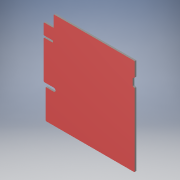
# Autodesk Inventor part: Avionics_PCB
Saved by Autodesk Inventor 2018 (Build 220112000, 112)
## iProperties
Created: 2018-01-15
Part Number: Avionics_PCB
Material: Epoxy Resin
Document SubType Name: Modeling
Designer: Bradley
Density: 1.14 g/cm^3
Appearance: Smooth - Medium Gray
Mass: 15.4834 g
Surface Area: 175.95 cm^2
Volume: 13.582 cm^3
Author: Bradley
Revision Number: 3.1
Autodesk Inventor part; units mm, degrees
ref_plane "XZ Plane" through (0, 0, 0) normal (0, 1, 0) x (-1, 0, 0)
ref_plane "XY Plane" through (0, 0, 0) normal (0, 0, 1) x (1, 0, 0)
sketch "Sketch1" plane through (0, 0, 0) normal (0, 0, 1) x (1, 0, 0)
  line L0 (0, 36.15) -> (10, 36.15)
  line L1 (10, 36.15) -> (10, 47.9)
  line L2 (10, 47.9) -> (90.4, 47.9)
  line L3 (90.4, 47.9) -> (90.4, -47.9)
  line L4 (90.4, -47.9) -> (2, -47.9)
  line L5 (10, -15.15) -> (0, -15.15)
  line L6 (-5.5, 48) -> (90.5, 48) construction
  line L7 (90.5, 48) -> (90.5, -48) construction
  line L8 (90.5, -48) -> (-5.5, -48) construction
  line L9 (-5.5, -48) -> (-5.5, 48) construction
  line L10 (-5.4, 47.9) -> (-3.4, 47.9) construction
  line L11 (-3.4, 47.9) -> (-3.4, -47.9) construction
  line L12 (-3.4, -47.9) -> (-5.4, -47.9) construction
  line L13 (-5.4, -47.9) -> (-5.4, 47.9) construction
  line L14 (-3.4, 38.5) -> (7.85, 38.5) construction
  line L15 (7.85, 38.5) -> (7.85, -17.5) construction
  line L16 (7.85, -17.5) -> (-3.4, -17.5) construction
  line L17 (-3.4, -17.5) -> (-3.4, 38.5) construction
  line L18 (2, -47.9) -> (2, -18.65)
  line L19 (2, -18.65) -> (10, -18.65)
  arc A0 (10, -18.65) -> (10, -15.15) centre (10, -16.9) ccw
  line L20 (0, 24) -> (90.5, 24) construction
  circle A1 centre (-2.5, 47.1) radius 0.9 construction
  circle A2 centre (-0.7, 47.1) radius 0.9 construction
  circle A3 centre (1.1, 47.1) radius 0.9 construction
  circle A4 centre (2.9, 47.1) radius 0.9 construction
  circle A5 centre (4.7, 47.1) radius 0.9 construction
  circle A6 centre (6.5, 47.1) radius 0.9 construction
  circle A7 centre (8.3, 47.1) radius 0.9 construction
  circle A8 centre (-2.5, 45.3) radius 0.9 construction
  circle A9 centre (-0.7, 45.3) radius 0.9 construction
  circle A10 centre (1.1, 45.3) radius 0.9 construction
  circle A11 centre (2.9, 45.3) radius 0.9 construction
  circle A12 centre (4.7, 45.3) radius 0.9 construction
  circle A13 centre (6.5, 45.3) radius 0.9 construction
  circle A14 centre (8.3, 45.3) radius 0.9 construction
  circle A15 centre (-2.5, 43.5) radius 0.9 construction
  circle A16 centre (-0.7, 43.5) radius 0.9 construction
  circle A17 centre (1.1, 43.5) radius 0.9 construction
  circle A18 centre (2.9, 43.5) radius 0.9 construction
  circle A19 centre (4.7, 43.5) radius 0.9 construction
  circle A20 centre (6.5, 43.5) radius 0.9 construction
  circle A21 centre (8.3, 43.5) radius 0.9 construction
  circle A22 centre (-2.5, 41.7) radius 0.9 construction
  circle A23 centre (-0.7, 41.7) radius 0.9 construction
  circle A24 centre (1.1, 41.7) radius 0.9 construction
  circle A25 centre (2.9, 41.7) radius 0.9 construction
  circle A26 centre (4.7, 41.7) radius 0.9 construction
  circle A27 centre (6.5, 41.7) radius 0.9 construction
  circle A28 centre (8.3, 41.7) radius 0.9 construction
  circle A29 centre (-2.5, 39.9) radius 0.9 construction
  circle A30 centre (-0.7, 39.9) radius 0.9 construction
  circle A31 centre (1.1, 39.9) radius 0.9 construction
  circle A32 centre (2.9, 39.9) radius 0.9 construction
  circle A33 centre (4.7, 39.9) radius 0.9 construction
  circle A34 centre (6.5, 39.9) radius 0.9 construction
  circle A35 centre (8.3, 39.9) radius 0.9 construction
  line L21 (0, 36.15) -> (0, 24.95)
  line L22 (0, 24.95) -> (8.4, 24.95)
  arc A36 (8.4, 23.05) -> (8.4, 24.95) centre (8.4, 24) ccw
  line L23 (8.4, 23.05) -> (0, 23.05)
  line L24 (0, 23.05) -> (0, -15.15)
  point P0 (0, 0)
  point P1 (-5.5, 0)
  point P2 (90.4, 0)
  point P3 (90.5, 0)
  dimension "d0" = 51.3
  dimension "d1" = 95.8
  dimension "d3" = 10
  dimension "d20" = 96
  dimension "d21" = 96
  dimension "d22" = 0.1
  dimension "d23" = 0.1
  dimension "d24" = 2
  dimension "d25" = 0.1
  dimension "d28" = 11.25
  dimension "d29" = 56
  dimension "d31" = 9.5
  dimension "d32" = 30.5
  dimension "d34" = 3.5
  dimension "d35" = 12.15
  dimension "d36" = 39.15
  dimension "d37" = 14.5
  dimension "d38" = 1.15
  dimension "d39" = 1.8
  dimension "d42" = 1.8
  dimension "d45" = 1.8
  dimension "d48" = 2
  dimension "d49" = 3.4
  dimension "d50" = 1.9
  dimension "d51" = 8.4
  dimension "d52" = 24
  constraints: 50 end point, 37 centre point, 11 perpendicular, 7 parallel, 6 point on line, 6 tangent, 5 horizontal, 4 point on circle, 3 midpoint, 3 vertical, 2 collinear, 2 horizontal alignment, 68 other
  measures "d0" distance of L5.end L0.start
  measures "d1" distance of L2.end L3.end
  measures "d3" distance of L0.start L0.end
  measures "d20" distance of L6.start L6.end
  measures "d21" distance of L8.end L6.start
  measures "d22" distance between parallel lines of L2 L6
  measures "d23" distance between parallel lines of L7 L3
  measures "d24" distance between parallel lines of L13 L11
  measures "d25" distance between parallel lines of L13 L9
  measures "d28" distance of L15.end L16.end
  measures "d29" distance of L14.end L15.end
  measures "d31" distance between parallel lines of L14 L6
  measures "d32" distance between parallel lines of L8 L16
  measures "d34" distance between parallel lines of L5 L19
  measures "d35" distance between parallel lines of L20 L0
  measures "d36" distance between parallel lines of L5 L20
  measures "d37" distance between parallel lines of L20 L14
  measures "d38" distance between parallel lines of L19 L16
  measures "d39" diameter of A1
  measures "d42" distance of A1.centre A2.centre
  measures "d45" distance of A1.centre A8.centre
  measures "d48" distance between parallel lines of L18 L24
  measures "d49" distance between parallel lines of L24 L11
  measures "d50" distance between parallel lines of L23 L22
  measures "d51" distance of L21.end L22.end
  measures "d52" distance from line of point (0, 0) L20
extrude "Extrusion1" add sketch "Sketch1" along normal mid plane 1.6
chamfer "Chamfer1" distance 0.5 angle 45 4 edges at (0, 36.15, 0) (0, 24.95, 0) (0, 23.05, 0) (0, -15.15, 0)
fillet "Fillet1" radius 0.5 6 edges at (10, 36.15, 0) (10, 47.9, 0) (90.4, 47.9, 0) (90.4, -47.9, 0) (2, -47.9, 0) (2, -18.65, 0)
sketch "Sketch16" plane through (0, 0, 0.8) normal (0, 0, 1) x (1, 0, 0)
  arc A0 (2.5, -18.65) -> (2, -19.15) centre (2.5, -19.15) ccw projected
  line L0 (2, -19.15) -> (2, -47.4) projected
  arc A1 (2, -47.4) -> (2.5, -47.9) centre (2.5, -47.4) ccw projected
  line L1 (2.5, -47.9) -> (89.9, -47.9) projected
  arc A2 (89.9, -47.9) -> (90.4, -47.4) centre (89.9, -47.4) ccw projected
  line L2 (90.4, -47.4) -> (90.4, 47.4) projected
  arc A3 (90.4, 47.4) -> (89.9, 47.9) centre (89.9, 47.4) ccw projected
  line L3 (89.9, 47.9) -> (10.5, 47.9) projected
  arc A4 (10.5, 47.9) -> (10, 47.4) centre (10.5, 47.4) ccw projected
  line L4 (10, 47.4) -> (10, 36.65) projected
  arc A5 (9.5, 36.15) -> (10, 36.65) centre (9.5, 36.65) ccw projected
  line L5 (9.5, 36.15) -> (0.5, 36.15) projected
  line L6 (0, 35.65) -> (0.5, 36.15) projected
  line L7 (0, 35.65) -> (0, 25.45) projected
  line L8 (0.5, 24.95) -> (0, 25.45) projected
  line L9 (0.5, 24.95) -> (8.4, 24.95) projected
  arc A6 (8.4, 23.05) -> (8.4, 24.95) centre (8.4, 24) ccw projected
  line L10 (8.4, 23.05) -> (0.5, 23.05) projected
  line L11 (0, 22.55) -> (0.5, 23.05) projected
  line L12 (0, 22.55) -> (0, -14.65) projected
  line L13 (0.5, -15.15) -> (0, -14.65) projected
  line L14 (0.5, -15.15) -> (10, -15.15) projected
  arc A7 (10, -18.65) -> (10, -15.15) centre (10, -16.9) ccw projected
  line L15 (10, -18.65) -> (2.5, -18.65) projected
  line L16 (90.4, -47.4) -> (90.4, 47.4) projected
  arc A8 (89.4, 33) -> (90.4, 34) centre (89.4, 34) ccw
  arc A9 (89.4, 33) -> (88.4, 32) centre (89.4, 32) ccw
  arc A10 (88.4, 26) -> (89.4, 25) centre (89.4, 26) ccw
  arc A11 (90.4, 24) -> (89.4, 25) centre (89.4, 24) ccw
  line L17 (88.4, 32) -> (88.4, 26)
  line L18 (88.4, 29) -> (90.4, 29) construction
  point P0 (0, 0)
  dimension "d145" = 1
  dimension "d146" = 29
  dimension "d147" = 8
  dimension "d148" = 34
  constraints: 8 point on circle, 6 tangent, 4 centre point, 4 end point, 3 equal radius, 3 point on line, 1 midpoint, 1 perpendicular, 1 vertical, 1 vertical alignment
  measures "d145" radius of A11
  measures "d146" distance from line of L18 point (0, 0)
  measures "d147" distance of A10.end A8.start
  measures "d148" vertical distance of point (0, 0) A8.end
extrude "Extrusion6" cut sketch "Sketch16" against normal through all contours A11 A10 L17 A9 A8 L2
ref_plane "Work Plane1" through (4, 0, 0) normal (1, 0, 0) x (0, 1, 0)
sketch "Sketch17" plane through (4, 0, 0) normal (1, 0, 0) x (0, 1, 0)
  line L0 (-19.15, -0.8) -> (-19.15, 0.8) projected
  line L1 (-47.4, -0.8) -> (-19.15, -0.8) projected
  line L2 (-47.4, 0.8) -> (-47.4, -0.8) projected
  line L3 (-19.15, 0.8) -> (-47.4, 0.8) projected
  point P0 (0, 0)
  point P1 (-42, 1.8)
  point P2 (-41, 1.8)
  point P3 (-40, 1.8)
  point P4 (-39, 1.8)
  point P5 (-42, 2.8)
  point P6 (-41, 2.8)
  point P7 (-40, 2.8)
  point P8 (-39, 2.8)
  point P9 (-42, 3.8)
  point P10 (-41, 3.8)
  point P11 (-40, 3.8)
  point P12 (-39, 3.8)
  point P13 (-42, 4.8)
  point P14 (-41, 4.8)
  point P15 (-40, 4.8)
  point P16 (-39, 4.8)
  dimension "d154" = 1
  dimension "d157" = 1
  dimension "d160" = 42
  dimension "d161" = 1
  constraints: 1 horizontal, 1 vertical, 15 other
  measures "d154" distance of point (-42, 1.8) point (-41, 1.8)
  measures "d157" distance of point (-42, 1.8) point (-42, 2.8)
  measures "d160" horizontal distance of point (-42, 1.8) point (0, 0)
  measures "d161" distance from line of L3 point (-42, 1.8)
sketch "Sketch18" plane through (0, 0, 0) normal (0, 0, 1) x (1, 0, 0)
  arc A0 (90.4, 24) -> (89.4, 25) centre (89.4, 24) ccw projected
  arc A1 (88.4, 26) -> (89.4, 25) centre (89.4, 26) ccw projected
  line L0 (88.4, 26) -> (88.4, 32) projected
  arc A2 (89.4, 33) -> (88.4, 32) centre (89.4, 32) ccw projected
  arc A3 (89.4, 33) -> (90.4, 34) centre (89.4, 34) ccw projected
  line L1 (90.4, 34) -> (90.4, 47.4) projected
  arc A4 (90.4, 47.4) -> (89.9, 47.9) centre (89.9, 47.4) ccw projected
  line L2 (89.9, 47.9) -> (10.5, 47.9) projected
  arc A5 (10.5, 47.9) -> (10, 47.4) centre (10.5, 47.4) ccw projected
  line L3 (10, 47.4) -> (10, 36.65) projected
  arc A6 (9.5, 36.15) -> (10, 36.65) centre (9.5, 36.65) ccw projected
  line L4 (9.5, 36.15) -> (0.5, 36.15) projected
  line L5 (0, 35.65) -> (0.5, 36.15) projected
  line L6 (0, 35.65) -> (0, 25.45) projected
  line L7 (0.5, 24.95) -> (0, 25.45) projected
  line L8 (0.5, 24.95) -> (8.4, 24.95) projected
  arc A7 (8.4, 23.05) -> (8.4, 24.95) centre (8.4, 24) ccw projected
  line L9 (8.4, 23.05) -> (0.5, 23.05) projected
  line L10 (0, 22.55) -> (0.5, 23.05) projected
  line L11 (0, 22.55) -> (0, -14.65) projected
  line L12 (0.5, -15.15) -> (0, -14.65) projected
  line L13 (0.5, -15.15) -> (10, -15.15) projected
  arc A8 (10, -18.65) -> (10, -15.15) centre (10, -16.9) ccw projected
  line L14 (10, -18.65) -> (2.5, -18.65) projected
  arc A9 (2.5, -18.65) -> (2, -19.15) centre (2.5, -19.15) ccw projected
  line L15 (2, -19.15) -> (2, -47.4) projected
  arc A10 (2, -47.4) -> (2.5, -47.9) centre (2.5, -47.4) ccw projected
  line L16 (2.5, -47.9) -> (89.9, -47.9) projected
  arc A11 (89.9, -47.9) -> (90.4, -47.4) centre (89.9, -47.4) ccw projected
  line L17 (90.4, -47.4) -> (90.4, 24) projected
  point P0 (0, 0)
  point P1 (1.5, -44.9)
  point P2 (0.5, -44.9)
  point P3 (1.5, -43.9)
  point P4 (0.5, -43.9)
  point P5 (1.5, -42.9)
  point P6 (0.5, -42.9)
  point P7 (1.5, -41.9)
  point P8 (0.5, -41.9)
  point P9 (1.5, -40.9)
  point P10 (0.5, -40.9)
  point P11 (1.5, -39.9)
  point P12 (0.5, -39.9)
  point P13 (1.5, -38.9)
  point P14 (0.5, -38.9)
  point P15 (1.5, -37.9)
  point P16 (0.5, -37.9)
  point P17 (1.5, -36.9)
  point P18 (0.5, -36.9)
  point P19 (1.5, -35.9)
  point P20 (0.5, -35.9)
  point P21 (1.5, -34.9)
  point P22 (0.5, -34.9)
  point P23 (1.5, -33.9)
  point P24 (0.5, -33.9)
  point P25 (1.5, -32.9)
  point P26 (0.5, -32.9)
  point P27 (1.5, -31.9)
  point P28 (0.5, -31.9)
  point P29 (1.5, -30.9)
  point P30 (0.5, -30.9)
  point P31 (1.5, -29.9)
  point P32 (0.5, -29.9)
  point P33 (1.5, -28.9)
  point P34 (0.5, -28.9)
  point P35 (1.5, -27.9)
  point P36 (0.5, -27.9)
  point P37 (1.5, -26.9)
  point P38 (0.5, -26.9)
  point P39 (1.5, -25.9)
  point P40 (0.5, -25.9)
  point P41 (1.5, -24.9)
  point P42 (0.5, -24.9)
  point P43 (1.5, -23.9)
  point P44 (0.5, -23.9)
  point P45 (1.5, -22.9)
  point P46 (0.5, -22.9)
  point P47 (1.5, -21.9)
  point P48 (0.5, -21.9)
  point P49 (1.5, -20.9)
  point P50 (0.5, -20.9)
  point P51 (9.5, 37.9)
  point P52 (9.5, 38.9)
  point P53 (9.5, 39.9)
  point P54 (9.5, 40.9)
  point P55 (9.5, 41.9)
  point P56 (9.5, 42.9)
  point P57 (9.5, 43.9)
  point P58 (8.5, 37.9)
  point P59 (8.5, 38.9)
  point P60 (8.5, 39.9)
  point P61 (8.5, 40.9)
  point P62 (8.5, 41.9)
  point P63 (8.5, 42.9)
  point P64 (8.5, 43.9)
  point P65 (7.5, 37.9)
  point P66 (7.5, 38.9)
  point P67 (7.5, 39.9)
  point P68 (7.5, 40.9)
  point P69 (7.5, 41.9)
  point P70 (7.5, 42.9)
  point P71 (7.5, 43.9)
  point P72 (6.5, 37.9)
  point P73 (6.5, 38.9)
  point P74 (6.5, 39.9)
  point P75 (6.5, 40.9)
  point P76 (6.5, 41.9)
  point P77 (6.5, 42.9)
  point P78 (6.5, 43.9)
  dimension "d164" = 1
  dimension "d167" = 1
  dimension "d170" = 0.5
  dimension "d171" = 3
  dimension "d172" = 0.5
  dimension "d173" = 10
  dimension "d176" = 1
  dimension "d179" = 1
  constraints: 2 horizontal, 2 vertical, 76 other
  measures "d164" distance of point (1.5, -44.9) point (0.5, -44.9)
  measures "d167" distance of point (1.5, -44.9) point (1.5, -43.9)
  measures "d170" distance from line of L15 point (1.5, -44.9)
  measures "d171" distance from line of L16 point (1.5, -44.9)
  measures "d172" distance from line of point (9.5, 37.9) L3
  measures "d173" distance from line of point (9.5, 37.9) L2
  measures "d176" distance of point (9.5, 37.9) point (9.5, 38.9)
  measures "d179" distance of point (9.5, 37.9) point (8.5, 37.9)
equation "\"d23\" = d22"
equation "\"d25\" = d22"
equation "\"d42\" = d39"
equation "\"d45\" = d39"
body "Solid1"
